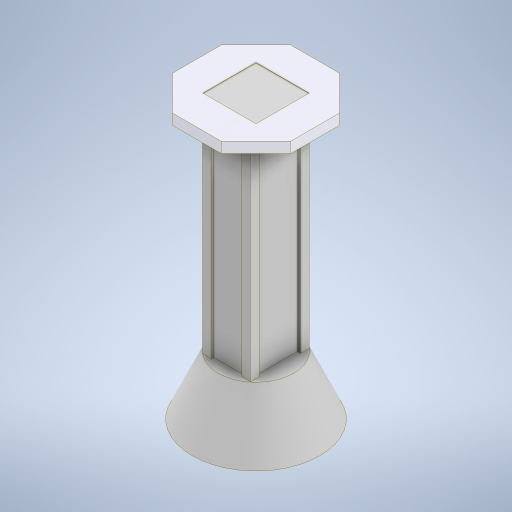
# Autodesk Inventor part: 盤子上布丁
Saved by Autodesk Inventor 2024.2 (Build 282272000, 272)
## iProperties
Created: 2024-06-04
Part Number: 盤子上布丁
Material: 一般
Document SubType Name: Modeling
Designer: sohil
Density: 1 g/cm^3
Appearance: 銀色
Author: sohil
Autodesk Inventor part; units mm, degrees
ref_plane "YZ Plane" through (0, 0, 0) normal (1, 0, 0) x (0, 1, 0)
ref_plane "XZ Plane" through (0, 0, 0) normal (0, 1, 0) x (-1, 0, 0)
ref_plane "XY Plane" through (0, 0, 0) normal (0, 0, 1) x (1, 0, 0)
sketch "草圖1" plane through (0, 0, 0) normal (0, 1, 0) x (-1, 0, 0)
  circle A0 centre (0, 0.3443) radius 12
  point P0 (0, 0)
  dimension "d0" = 24
  constraints: 1 centre point
  measures "d0" diameter of A0
extrude "擠出1" add sketch "草圖1" along normal blind 11
draft "面拔模1" angle 24 pull direction (0, 1, 0) faces at (-11.8446, 7.3333, -1.5807) fixed edges at (12, 0, 0.3443)
sketch "草圖2" plane through (0, 11, 0.3443) normal (0, 1, 0) x (1, 0, 0)
  line L0 (-4.5495, -3.8466) -> (-2.9152, -3.8466)
  line L1 (-2.9152, -3.8466) -> (-2.9152, -5.5016)
  line L2 (-2.9152, -5.5016) -> (-4.5495, -5.5016)
  line L3 (-4.5495, -5.5016) -> (-4.5495, -3.8466)
  circle A0 centre (0, 0) radius 7.1025 projected
  line L4 (-4.5495, 5.4541) -> (-2.9152, 5.4541)
  line L5 (-2.9152, 5.4541) -> (-2.9152, 3.8283)
  line L6 (-2.9152, 3.8283) -> (-4.5495, 3.8283)
  line L7 (-4.5495, 3.8283) -> (-4.5495, 5.4541)
  line L8 (4.5495, 5.4541) -> (2.8978, 5.4541)
  line L9 (2.8978, 5.4541) -> (2.8978, 3.8283)
  line L10 (2.8978, 3.8283) -> (4.5495, 3.8283)
  line L11 (4.5495, 3.8283) -> (4.5495, 5.4541)
  line L12 (4.492, -5.5016) -> (2.862, -5.5016)
  line L13 (2.862, -5.5016) -> (2.862, -3.8466)
  line L14 (2.862, -3.8466) -> (4.492, -3.8466)
  line L15 (4.492, -3.8466) -> (4.492, -5.5016)
  line L16 (-3.9212, 3.8283) -> (-3.9212, -3.8466)
  line L17 (-2.9152, -5.0387) -> (2.862, -5.0387)
  line L18 (3.9473, -3.8466) -> (3.9473, 3.8283)
  line L19 (2.8978, 4.9975) -> (-2.9152, 4.9975)
  point P0 (0, 0.3443)
  dimension "d4" = 1.63
  constraints: 40 end point, 12 point on line, 8 parallel, 8 perpendicular, 4 horizontal, 3 point on circle
  measures "d4" distance of L13.end L14.end
extrude "擠出2" add sketch "草圖2" along normal blind 40 contours L0 L1 L2 A0 L3 | L16 L6 L5 L19 L9 L10 L18 L14 L13 L17 L1 L0 | A0 L2 L3 | L6 L7 L4 L5 | L11 L10 L9 L8 | L12 L13 L14 L15
sketch "草圖3" plane through (0, 51, 0.3443) normal (0, 1, 0) x (1, 0, 0)
  circle A0 centre (0, 0) radius 12 projected
  line L0 (-4.5956, 11.0851) -> (4.5888, 11.088)
  line L1 (4.5888, 11.088) -> (11.0851, 4.5956)
  line L2 (11.0851, 4.5956) -> (11.088, -4.5888)
  line L3 (11.088, -4.5888) -> (4.5956, -11.0851)
  line L4 (4.5956, -11.0851) -> (-4.5888, -11.088)
  line L5 (-4.5888, -11.088) -> (-11.0851, -4.5956)
  line L6 (-11.0851, -4.5956) -> (-11.088, 4.5888)
  line L7 (-11.088, 4.5888) -> (-4.5956, 11.0851)
  constraints: 16 end point, 19 other
extrude "擠出3" add sketch "草圖3" along normal blind 2 contours L2 L3 L4 L5 L6 L7 L0 L1
sketch "草圖4" plane through (0, 53, 0.3443) normal (0, 1, 0) x (1, 0, 0)
  line L0 (5, -5) -> (5, 5)
  line L1 (5, 5) -> (-5, 5)
  line L2 (-5, 5) -> (-5, -5)
  line L3 (-5, -5) -> (5, -5)
  line L4 (5, -5) -> (-5, 5) construction
  line L5 (5, 5) -> (-5, -5) construction
  point P0 (0, 0.3443)
  point P1 (0, 0)
  dimension "d9" = 10
  dimension "d10" = 10
  constraints: 12 end point, 2 midpoint, 2 parallel, 1 perpendicular, 1 vertical
  measures "d9" distance of L0.start L0.end
  measures "d10" distance of L1.end L0.end
extrude "擠出4" cut sketch "草圖4" against normal blind 0.1
